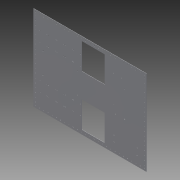
# Autodesk Inventor part: baseplate archive 2
Saved by Autodesk Inventor 2014 SP1 (Build 180222100, 222)
## iProperties
Created: 2014-01-05
Part Number: baseplate archive 2
Material: Aluminum 6061
Document SubType Name: Sheet Metal
Designer: Arpan
Density: 2.71 g/cm^3
Sheet Metal Rule: Default
Appearance: Aluminum - Flat
Mass: 1326.97 g
Surface Area: 6245.09 cm^2
Volume: 489.657 cm^3
Author: Arpan
Autodesk Inventor part; units mm, degrees
ref_plane "YZ Plane" through (0, 0, 0) normal (1, 0, 0) x (0, 1, 0)
ref_plane "XZ Plane" through (0, 0, 0) normal (0, 1, 0) x (-1, 0, 0)
ref_plane "XY Plane" through (0, 0, 0) normal (0, 0, 1) x (1, 0, 0)
sketch "Sketch1" plane through (0, 0, 0) normal (0, 0, 1) x (1, 0, 0)
  line L0 (0, 0) -> (-685.8, 0)
  line L1 (-685.8, 0) -> (-685.8, 516.255)
  line L2 (-685.8, 516.255) -> (0, 516.255)
  line L3 (0, 516.255) -> (0, 0)
  dimension "d0" = 685.8
  dimension "d1" = 516.255
  measures "d0" distance of L1.end L2.end
  measures "d1" distance of L2.end L0.start
extrude "Plate1" add sketch "Sketch1" along normal blind 1.5875
sketch "Sketch4" plane through (0, 0, 1.5875) normal (0, 0, 1) x (1, 0, 0)
  circle A0 centre (-673.1, 503.555) radius 2.0828 projected
  circle A1 centre (-673.1, 12.7) radius 2.0828 projected
extrude "Cut3" cut sketch "Sketch4" against normal blind 1.5875
pattern_linear "Rectangular Pattern2" count 27 spacing 25.4 along (1, 0, 0) of "Cut3"
sketch "Sketch2" plane through (0, 0, 1.5875) normal (0, 0, 1) x (1, 0, 0)
  line L0 (0, 0) -> (-685.8, 0) projected
  line L1 (-685.8, 516.255) -> (0, 516.255) projected
  line L2 (-342.9, 516.255) -> (-392.43, 516.255)
  line L3 (-392.43, 516.255) -> (-392.43, 332.105)
  line L4 (-392.43, 332.105) -> (-252.73, 332.105)
  line L5 (-252.73, 332.105) -> (-252.73, 516.255)
  line L6 (-392.43, 0) -> (-392.43, 184.15)
  line L7 (-392.43, 184.15) -> (-252.73, 184.15)
  line L8 (-252.73, 184.15) -> (-252.73, 0)
  line L9 (-392.43, 0) -> (-392.43, 25.4)
  line L10 (-392.43, 25.4) -> (-252.73, 25.4)
  line L11 (-252.73, 516.255) -> (-252.73, 490.855)
  line L12 (-252.73, 490.855) -> (-392.43, 490.855)
  line L13 (-685.8, 0) -> (-685.8, 516.255) projected
  dimension "d4" = 184.15
  dimension "d5" = 139.7
  dimension "d6" = 184.15
  dimension "d23" = 25.4
  dimension "d24" = 25.4
  dimension "d78" = 293.37
  dimension "d79" = 139.7
  dimension "d80" = 293.37
  constraints: 22 end point, 8 point on line, 6 perpendicular, 2 parallel, 1 midpoint
  measures "d4" distance of L2.end L3.end
  measures "d5" distance of L3.end L4.end
  measures "d6" distance of L6.start L6.end
  measures "d23" distance of L6.start L9.end
  measures "d24" distance of L5.end L11.end
  measures "d78" distance between parallel lines of L13 L6
  measures "d79" distance between parallel lines of L8 L6
  measures "d80" distance between parallel lines of L13 L3
extrude "Cut6" cut sketch "Sketch2" against normal blind 1.5875 contours L10 L6 L7 L8 | L12 L5 L4 L3
sketch "Sketch12" plane through (0, 0, 1.5875) normal (0, 0, 1) x (1, 0, 0)
  arc A0 (-673.1762, 31.5962) -> (-673.1762, 27.4588) centre (-673.1, 29.5275) ccw projected
  arc A1 (-673.0238, 27.4588) -> (-673.0238, 31.5962) centre (-673.1, 29.5275) ccw projected
  circle A2 centre (-673.1, 29.5275) radius 2.0701
  constraints: 1 centre point, 1 coincident, 1 concentric
extrude "Cut8" cut sketch "Sketch12" against normal blind 1.5875
pattern_linear "Rectangular Pattern5" count 19 spacing 25.4 along (0, 1, 0) count 2 spacing 660.4 along (1, 0, 0) of "Cut8"
sketch "Sketch16" plane through (0, 0, 1.5875) normal (0, 0, 1) x (1, 0, 0)
  line L0 (-685.8, 0) -> (-685.8, 516.255) projected
  line L1 (0, 516.255) -> (0, 0) projected
  circle A0 centre (-602.8344, 420.0249) radius 2.1723 projected
  circle A1 centre (-644.6428, 357.8965) radius 2.1989 projected
  circle A2 centre (-593.5881, 357.8965) radius 2.1989 projected
  circle A3 centre (-551.7797, 420.0249) radius 2.1723 projected
  circle A4 centre (-542.5208, 357.8965) radius 2.1989 projected
  circle A5 centre (-500.7124, 420.0249) radius 2.1723 projected
  circle A6 centre (-449.633, 420.0249) radius 2.1723 projected
  circle A7 centre (-491.4414, 357.8965) radius 2.1989 projected
  circle A8 centre (-440.3741, 357.8965) radius 2.1989 projected
  circle A9 centre (-398.5657, 420.0249) radius 2.1723 projected
  circle A10 centre (-417.8895, 321.6304) radius 3.2639 projected
  circle A11 centre (-417.8895, 194.6304) radius 3.2639 projected
  circle A12 centre (-627.4395, 321.6304) radius 3.2639 projected
  circle A13 centre (-627.4395, 194.6304) radius 3.2639 projected
  circle A14 centre (-644.6428, 96.019) radius 2.1989 projected
  circle A15 centre (-602.8344, 158.1474) radius 2.1723 projected
  circle A16 centre (-593.5881, 96.019) radius 2.1989 projected
  circle A17 centre (-551.7797, 158.1474) radius 2.1723 projected
  circle A18 centre (-542.5208, 96.019) radius 2.1989 projected
  circle A19 centre (-500.7124, 158.1474) radius 2.1723 projected
  circle A20 centre (-449.633, 158.1474) radius 2.1723 projected
  circle A21 centre (-491.4414, 96.019) radius 2.1989 projected
  circle A22 centre (-440.3741, 96.019) radius 2.1989 projected
  circle A23 centre (-398.5657, 158.1474) radius 2.1723 projected
  line L2 (-685.8, 258.1275) -> (0, 258.1275)
  circle A24 centre (-602.8344, 96.2301) radius 2.1723
  circle A25 centre (-644.6428, 158.3585) radius 2.1989
  circle A26 centre (-593.5881, 158.3585) radius 2.1989
  circle A27 centre (-551.7797, 96.2301) radius 2.1723
  circle A28 centre (-542.5208, 158.3585) radius 2.1989
  circle A29 centre (-500.7124, 96.2301) radius 2.1723
  circle A30 centre (-449.633, 96.2301) radius 2.1723
  circle A31 centre (-491.4414, 158.3585) radius 2.1989
  circle A32 centre (-440.3741, 158.3585) radius 2.1989
  circle A33 centre (-398.5657, 96.2301) radius 2.1723
  circle A34 centre (-644.6428, 420.236) radius 2.1989
  circle A35 centre (-602.8344, 358.1076) radius 2.1723
  circle A36 centre (-593.5881, 420.236) radius 2.1989
  circle A37 centre (-551.7797, 358.1076) radius 2.1723
  circle A38 centre (-542.5208, 420.236) radius 2.1989
  circle A39 centre (-500.7124, 358.1076) radius 2.1723
  circle A40 centre (-449.633, 358.1076) radius 2.1723
  circle A41 centre (-491.4414, 420.236) radius 2.1989
  circle A42 centre (-440.3741, 420.236) radius 2.1989
  circle A43 centre (-398.5657, 358.1076) radius 2.1723
  circle A44 centre (-133.294, 368.9594) radius 2.2479 projected
  circle A45 centre (-194.254, 368.9594) radius 1.5457 projected
  circle A46 centre (-196.794, 254.6594) radius 2.2655 projected
  circle A47 centre (-198.3647, 418.811) radius 2.5119 projected
  circle A48 centre (-151.1207, 418.811) radius 2.5119 projected
  circle A49 centre (-187.6385, 209.9079) radius 3.5177 projected
  circle A50 centre (-131.6773, 209.9079) radius 3.5177 projected
  circle A51 centre (-197.0948, 95.631) radius 2.4116 projected
  circle A52 centre (-197.0948, 59.563) radius 2.4116 projected
  circle A53 centre (-57.15, 57.15) radius 2.4116 projected
  circle A54 centre (-57.15, 98.044) radius 2.4116 projected
  constraints: 20 symmetric about line, 2 end point, 2 midpoint, 20 other
extrude "Cut9" cut sketch "Sketch16" against normal blind 1.5875 contours A0 | A1 | A2 | A3 | A4 | A5 | A6 | A7 | A8 | A9 | A10 | A11 | A12 | A13 | A14 | A15 | A16 | A17 | A18 | A19 | A20 | A21 | A22 | A23 | A24 | A25 | A26 | A27 | A28 | A29 | A30 | A31 | A32 | A33 | A34 | A35 | A36 | A37 | A38 | A39 | A40 | A41 | A42 | A43 | A44 | A46 | A47 | A48 | A49 | A50 | A51 | A52 | A53 | A54
equation "\"d17\" = Thickness"
equation "\"d65\" = Thickness"
equation "\"BendRadius\" = Thickness"
equation "\"BendReliefWidth\" = Thickness"
equation "\"BendReliefDepth\" = 0.5 * Thickness"
equation "\"CornerReliefSize\" = 4 * Thickness"
equation "\"MinimumRemnant\" = 2 * Thickness"
equation "\"TransitionRadius\" = BendRadius"
equation "\"JacobiRadiusSize\" = Thickness"
equation "\"GapSize\" = Thickness"
equation "\"d2\" = BendRadius"
equation "\"Thickness\" = 1.5875"
body "Solid1"
